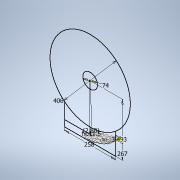
# Autodesk Inventor part: ArrayBracket
Saved by Autodesk Inventor 2022 (Build 260153070, 153G)
## iProperties
Created: 2021-11-12
Part Number: ArrayBracket
Material: Generic
Document SubType Name: Modeling
Designer: elmar
Density: 1 g/cm^3
Appearance: Default
Author: elmar
Autodesk Inventor part; units mm, degrees
ref_plane "YZ Plane" through (0, 0, 0) normal (1, 0, 0) x (0, 1, 0)
ref_plane "XZ Plane" through (0, 0, 0) normal (0, 1, 0) x (-1, 0, 0)
ref_plane "XY Plane" through (0, 0, 0) normal (0, 0, 1) x (1, 0, 0)
sketch "Sketch1" plane through (0, 0, 0) normal (0, 0, 1) x (1, 0, 0)
  circle A0 centre (0, 0) radius 203
  line L0 (-129, -156.741826) -> (-129, -267)
  line L1 (-129, -267) -> (129, -267)
  line L2 (129, -267) -> (129, -156.741826)
  circle A1 centre (0, 0) radius 37
  line L3 (0, -203) -> (0, -267)
  line L4 (0, -235) -> (-129, -235)
  line L5 (0, -235) -> (11.5, -235)
  dimension "d0" = 406
  dimension "d1" = 267
  dimension "d2" = 74
  dimension "d3" = 258
  dimension "d11" = 11.5
  dimension "HalfAngle" = 2.802
  constraints: 12 end point, 3 perpendicular, 3 point on circle, 2 centre point, 2 coincident, 2 midpoint, 2 vertical, 1 horizontal, 1 parallel, 1 point on line
  measures "d0" diameter of A0
  measures "d1" distance from line of L1 point (0, 0)
  measures "d2" diameter of A1
  measures "d3" distance of L0.end L1.end
  measures "d11" distance of L4.start L5.end
extrude "Extrusion1" add sketch "Sketch1" along normal blind 74 contours A1
ref_plane "Work Plane1" through (0, -235, 0) normal (0, -1, 0) x (-1, 0, 0)
sketch "Sketch2" plane through (0, -235, 0) normal (0, -1, 0) x (-1, 0, 0)
  line L0 (0, 13.279056) -> (11.5, 6.639528)
  line L1 (11.5, 6.639528) -> (11.5, -6.639528)
  line L2 (11.5, -6.639528) -> (0, -13.279056)
  line L3 (0, -13.279056) -> (-11.5, -6.639528)
  line L4 (-11.5, -6.639528) -> (-11.5, 6.639528)
  line L5 (-11.5, 6.639528) -> (0, 13.279056)
  point P0 (0, 0)
  point P1 (0, 0)
  dimension "d8" = 23
  constraints: 12 end point, 1 coincident, 1 vertical, 13 other
  measures "d8" distance between parallel lines of L1 L4
extrude "Extrusion2" add sketch "Sketch2" along normal blind 2 draft 2.8016 separate body
sketch "Sketch3" plane through (0, -235, 0) normal (0, 1, 0) x (1, 0, 0)
  line L0 (0, 0) -> (-5.798936, -10.044052)
  line L1 (-11.597872, -6.696035) -> (0, -13.392069)
  point P0 (-0.635, -1.099852)
  point P1 (-1.905, -3.299557)
  point P2 (-3.175, -5.499261)
  dimension "d16" = 1.27
  dimension "d17" = 2.54
  dimension "d18" = 2.54
  constraints: 3 point on line, 2 end point, 1 midpoint
  measures "d16" distance of L0.start point (-0.635, -1.1)
  measures "d17" distance of point (-0.635, -1.1) point (-1.905, -3.3)
  measures "d18" distance of point (-1.905, -3.3) point (-3.175, -5.499)
hole "Hole1" at (-1.905, -235, 3.299557) at (-0.635, -235, 1.099852) at (-3.175, -235, 5.499261) direction (0, -1, 0) diameter 1.27 end through all bodies 2
pattern_circular "Circular Pattern1" count 7 over 33.61921 about axis through (0, 0, -10) along (0, 0, 1) of "Extrusion2", "Hole1" bodies 2
ref_plane "Work Plane2" through (0, -235, -13.279056) normal (-0.0487035, 0.9952446, 0.0843569) x (0.8660254, 0, 0.5)
sketch "Sketch4" plane through (0, -235, -13.279056) normal (-0.0487035, 0.9952446, 0.0843569) x (0.8660254, 0, 0.5)
  line L0 (-0.047473, 22.972461) -> (13.215684, 22.999869)
  line L1 (13.215684, 22.999869) -> (19.870998, 11.527343)
  line L2 (19.870998, 11.527343) -> (13.263156, 0.027408)
  line L3 (13.263156, 0.027408) -> (0, 0)
  line L4 (0, 0) -> (-6.655315, 11.472526)
  line L5 (-6.655315, 11.472526) -> (-0.047473, 22.972461)
  point P0 (6.639528, 11.445313)
  point P1 (6.607842, 11.499935)
  point P2 (0, 0)
  constraints: 12 end point, 2 coincident, 13 other
extrude "Extrusion3" add sketch "Sketch4" against normal blind 2 draft 2.8016 separate body
sketch "Sketch5" plane through (0, -235, -13.279056) normal (-0.0487035, 0.9952446, 0.0843569) x (0.8660254, 0, 0.5)
  line L0 (6.639528, 11.445313) -> (6.639528, 17.795313)
  point P0 (6.639528, 15.255313)
  point P1 (6.639528, 12.715313)
  dimension "d29" = 2.54
  dimension "d30" = 2.54
  dimension "d125" = 1.27
  constraints: 3 end point, 2 point on line, 1 vertical
  measures "d29" distance of point (6.64, 15.255) L0.end
  measures "d30" distance of point (6.64, 12.715) point (6.64, 15.255)
  measures "d125" distance of L0.start point (6.64, 12.715)
hole "Hole2" at (14.605345, -233.266613, -25.2972) at (13.341384, -233.514027, -23.107956) at (12.077424, -233.76144, -20.918712) direction (0.0487035, -0.9952446, -0.0843569) diameter 1.27 end through all bodies 3
pattern_circular "Circular Pattern2" count 6 over 28.01601 about axis through (0, 0, -10) along (0, 0, 1) of "Extrusion3", "Hole2" bodies 3
mirror "Mirror1" about plane through (0, 0, 0) normal (0, 0, 1) of "Extrusion3", "Hole2", "Circular Pattern2" bodies 3
ref_plane "Work Plane3" through (120.404511, -201.83936, -33.384245) normal (0, 0, 1) x (-0.957271, -0.2891923, 0)
sketch "Sketch16" plane through (79.062498, -221.604675, -6.696035) normal (0.2891923, -0.957271, 0) x (0.957271, 0.2891923, 0)
  line L0 (-1.437872, 0.346035) -> (-21.757872, 0.346035)
  line L1 (-21.757872, 0.346035) -> (-21.757872, 13.046035)
  line L2 (-21.757872, 13.046035) -> (-1.437872, 13.046035)
  line L3 (-1.437872, 13.046035) -> (-1.437872, 0.346035)
  line L4 (-1.437872, 0.346035) -> (-21.757872, 13.046035) construction
  line L5 (-21.757872, 0.346035) -> (-1.437872, 13.046035) construction
  circle A0 centre (-21.757872, 13.046035) radius 1.2
  circle A1 centre (-1.437872, 13.046035) radius 1.2
  circle A2 centre (-21.757872, 0.346035) radius 1.2
  circle A3 centre (-1.437872, 0.346035) radius 1.2
  circle A4 centre (-12.232872, 7.795887) radius 0.635
  circle A5 centre (-14.772872, 12.195296) radius 0.635
  circle A6 centre (-13.502872, 9.995592) radius 0.635
  line L6 (0, 0) -> (-11.597872, -6.696035)
  line L7 (0, 13.392069) -> (0, 0)
  line L8 (-11.597872, 20.088104) -> (0, 13.392069)
  line L9 (-23.195745, 13.392069) -> (-11.597872, 20.088104)
  line L10 (-23.195745, 13.392069) -> (-23.195745, 0)
  line L11 (-11.597872, -6.696035) -> (-23.195745, 0)
  point P0 (-11.597872, 6.696035)
  dimension "d94" = 12.7
  dimension "d95" = 20.32
  dimension "d96" = 2.4
  constraints: 12 end point, 8 coincident, 4 centre point, 3 equal radius, 2 midpoint, 2 parallel, 1 horizontal, 1 perpendicular
  measures "d94" distance of L0.end L1.end
  measures "d95" distance of L1.end L2.end
  measures "d96" diameter of A0
extrude "Extrusion11" add sketch "Sketch16" along normal up to surface (2 mm away) contours A2 L11 L1 L0 | A2 L1 A0 L2 A1 L3 A3 L0 | L0 L1 A2 | L0 A3 L6 L11 A2 | A3 L3 L0 | L0 L3 A3 L6 | A2 L11 L10 L9 A0 L1 | L3 A1 L8 L7 L6 A3 | A0 L9 L2 L1 | L1 L2 A0 | A1 L2 L3 | L3 L2 A1 L8 | A0 L9 L8 A1 L2 | A4 | A5 | A6 bodies 2
extrude "Extrusion10" [suppressed]
hole "Hole5" at (67.960191, -224.958691, 0) direction (0.2891923, -0.957271, 0) diameter 10 end through all bodies 2
sketch "Sketch17" plane through (130.112642, -195.692872, -13.279056) normal (0.8328249, 0.5535212, 0.0041232) x (-0.0432166, 0.0724459, -0.9964356)
  line L0 (3.400357, -10) -> (-6.599643, -10)
  line L1 (-6.599643, -10) -> (-6.599643, 0)
  line L2 (-6.599643, 0) -> (3.400357, 0)
  line L3 (3.400357, 0) -> (3.400357, -10)
  line L4 (3.400357, -10) -> (-6.599643, 0) construction
  line L5 (-6.599643, -10) -> (3.400357, 0) construction
  line L6 (-20.024584, -0.311884) -> (-6.680249, -1.440247)
  line L7 (-6.568446, 0.557419) -> (-6.680249, -1.440247)
  line L8 (-6.568446, 0.557419) -> (-19.80017, 1.67626)
  line L9 (-19.80017, 1.67626) -> (-20.024584, -0.311884)
  line L10 (-6.568446, 0.557419) -> (-6.680249, -1.440247)
  line L11 (0, 0) -> (13.263185, 0)
  point P0 (6.568446, 235.283209)
  point P1 (-1.599643, -5)
  dimension "d108" = 10
  constraints: 12 end point, 2 midpoint, 2 parallel, 2 perpendicular, 1 collinear, 1 horizontal, 1 point on line
  measures "d108" distance of L0.end L1.end
extrude "Extrusion12" add sketch "Sketch17" along normal blind 5 contours L0 L1 L2 L3 bodies 3
ref_plane "Work Plane9" through (67.635469, -223.883813, 26.526539) normal (0.957271, 0.2891923, 0) x (0.2873565, -0.9511941, 0.1124989)
sketch "Sketch19" plane through (130.112642, -195.692872, -13.279056) normal (0.8328249, 0.5535212, 0.0041232) x (-0.0432166, 0.0724459, -0.9964356)
  line L0 (3.400357, -10) -> (3.400357, 0)
  line L1 (3.400357, 0) -> (-6.599643, 0)
  line L2 (-6.599643, 0) -> (-6.599643, -10)
  line L3 (-6.599643, -10) -> (3.400357, -10)
  circle A0 centre (-1.599643, -5) radius 5
  line L4 (3.400357, 0) -> (-6.599643, 0)
  line L5 (-4.763751, -4.732131) -> (-2.949715, -2.125868)
  line L6 (-2.949715, -2.125868) -> (0.214393, -2.393737)
  line L7 (0.214393, -2.393737) -> (1.564465, -5.267869)
  line L8 (1.564465, -5.267869) -> (-0.24957, -7.874132)
  line L9 (-0.24957, -7.874132) -> (-3.413678, -7.606263)
  line L10 (-3.413678, -7.606263) -> (-4.763751, -4.732131)
  line L11 (-6.744606, -1.436188) -> (-0.056507, -2.002393)
  point P0 (6.568446, 235.283209)
  dimension "d126" = 5.5
  constraints: 12 end point, 3 tangent, 1 centre point, 1 coincident, 1 parallel, 13 other
  measures "d126" distance between parallel lines of L6 L9
extrude "Extrusion13" cut sketch "Sketch19" along normal blind 2.4 contours L5 L6 L7 L8 L9 L10 bodies 3
hole "Hole8" at (132.941008, -199.957151, -12.106395) direction (0.8328249, 0.5535212, 0.0041232) diameter 3.4 end through all bodies 3 clearance for "Socket Head Cap Screw" size "M3" standard "Ansi Metric M Profile"
fillet "Fillet2" radius 3 2 edges at (137.9984, -203.084, -7.5352) (137.5662, -202.3595, -17.4995)
mirror "Mirror5" about plane through (67.635469, -223.883813, 26.526539) normal (0.957271, 0.2891923, 0) of "Extrusion12", "Extrusion13", "Fillet2", "Hole8" bodies 3
hole "Hole9" at (58.234317, -227.896884, -6.35) at (58.234317, -227.896884, 6.35) at (77.686064, -222.020497, 6.35) at (77.686064, -222.020497, -6.35) direction (0.2891923, -0.957271, 0) diameter 2.4 end through all countersink diameter 4.4 countersink angle 90 bodies 2 3 clearance for "Flat Head Machine Screw" size "M2" standard "Ansi Metric M Profile"
sketch "Sketch20" plane through (78.968807, -221.632979, 4.605179) normal (-0.2891923, 0.957271, 0) x (0.957271, 0.2891923, 0)
  arc A0 (-23.739382, 11.673629) -> (-23, 9.210358) centre (-21.66, 10.955179) ccw
  arc A1 (-20.409209, 12.765019) -> (-23.73072, 11.698227) centre (-21.66, 10.955179) ccw
  arc A2 (-23, 9.210358) -> (-20.480571, 12.812313) centre (-21.66, 10.955179) ccw
  arc A3 (-20.480571, -3.601955) -> (-23, 0) centre (-21.66, -1.744821) ccw
  arc A4 (-23, 0) -> (-23.739382, -2.463271) centre (-21.66, -1.744821) ccw
  arc A5 (-23.73072, -2.487869) -> (-20.409209, -3.554661) centre (-21.66, -1.744821) ccw
  arc A6 (0, 0) -> (-2.519429, -3.601955) centre (-1.34, -1.744821) ccw
  arc A7 (-2.519429, 12.812313) -> (0, 9.210358) centre (-1.34, 10.955179) ccw
  circle A8 centre (-21.66, -1.744821) radius 2.2
  circle A9 centre (-21.66, 10.955179) radius 2.2
  circle A10 centre (-1.34, -1.744821) radius 2.2
  line L0 (0, 9.210358) -> (0, 0)
  circle A11 centre (-1.34, 10.955179) radius 2.2
  point P0 (-11.5, 4.605179)
  point P1 (-2.519429, 12.812313)
  point P2 (0, 0)
  point P3 (-23.73072, -2.487869)
  constraints: 4 coincident, 12 other
extrude "Extrusion14" cut sketch "Sketch20" along normal through all bodies 2 3
sketch "Sketch21" plane through (134.276767, -192.925266, -13.25844) normal (0.8328249, 0.5535212, 0.0041232) x (-0.0432166, 0.0724459, -0.9964356)
  line L0 (-6.680249, -1.440247) -> (-0.055902, -2.00241)
  arc A0 (0.400357, -10) -> (3.400357, -7) centre (0.400357, -7) ccw
  line L1 (3.400357, -7) -> (3.400357, 0)
  line L2 (3.400357, 0) -> (-6.599643, 0)
  line L3 (-6.599643, 0) -> (-6.599643, -7)
  arc A1 (-6.599643, -7) -> (-3.599643, -10) centre (-3.599643, -7) ccw
  line L4 (-3.599643, -10) -> (0.400357, -10)
  circle A2 centre (-1.599643, -5) radius 1.7
  line L5 (-6.599643, 0) -> (-6.599643, -7)
  point P0 (6.568446, 235.283209)
  point P1 (-2.905048, -1.760623)
  dimension "d146" = 3.49251
  constraints: 1 point on line
  measures "d146" distance of A2.centre point (-2.905, -1.761)
equation "\"d11\" = 0.5 * d8"
equation "\"d10\" = HalfAngle"
equation "\"d14\" = 12 * HalfAngle"
equation "\"d27\" = HalfAngle"
equation "\"d39\" = 10 * HalfAngle"
body "Solid1"
body "Solid2"
body "Solid3"
